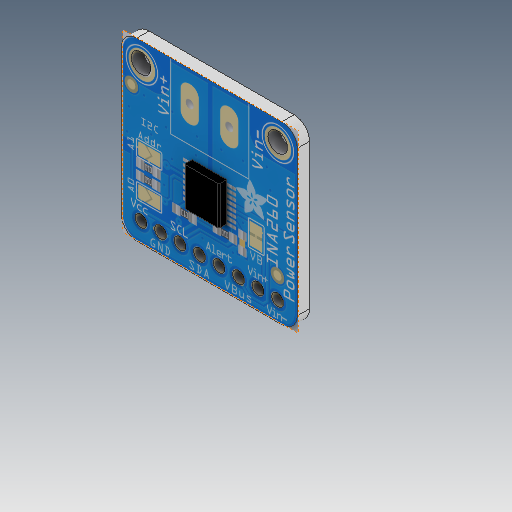
# Autodesk Inventor part: Adafruit_INA260
Saved by Autodesk Inventor 2020 (Build 240168000, 168)
## iProperties
Created: 2020-09-27
Part Number: Adafruit_INA260
Material: Generic
Document SubType Name: Modeling
Designer: DELL
Density: 1 g/cm^3
Appearance: Default
Author: DELL
Autodesk Inventor part; units mm, degrees
ref_plane "YZ Plane" through (0, 0, 0) normal (1, 0, 0) x (0, 1, 0)
ref_plane "XZ Plane" through (0, 0, 0) normal (0, 1, 0) x (-1, 0, 0)
ref_plane "XY Plane" through (0, 0, 0) normal (0, 0, 1) x (1, 0, 0)
sketch "Sketch1" plane through (0, 0, 0) normal (0, 0, 1) x (1, 0, 0)
  line L0 (11.43, -11.43) -> (-11.43, -11.43)
  line L1 (-11.43, -11.43) -> (-11.43, 11.43)
  line L2 (-11.43, 11.43) -> (11.43, 11.43)
  line L3 (11.43, 11.43) -> (11.43, -11.43)
  line L4 (11.43, -11.43) -> (-11.43, 11.43) construction
  line L5 (-11.43, -11.43) -> (11.43, 11.43) construction
  circle A0 centre (-8.89, 8.89) radius 1.27
  circle A1 centre (8.89, 8.89) radius 1.27
  line L6 (0, 11.43) -> (0, -11.43) construction
  circle A2 centre (-8.89, -8.89) radius 0.762
  circle A3 centre (-6.35, -8.89) radius 0.762
  circle A4 centre (-3.81, -8.89) radius 0.762
  circle A5 centre (-1.27, -8.89) radius 0.762
  circle A6 centre (1.27, -8.89) radius 0.762
  circle A7 centre (3.81, -8.89) radius 0.762
  circle A8 centre (6.35, -8.89) radius 0.762
  circle A9 centre (8.89, -8.89) radius 0.762
  point P0 (0, 0)
  dimension "d0" = 22.86
  dimension "d1" = 22.86
  dimension "d2" = 2.54
  dimension "d3" = 17.78
  dimension "d4" = 20.32
  dimension "d5" = 1.524
  dimension "d6" = 2.54
  dimension "d9" = 2.54
  constraints: 14 end point, 10 centre point, 4 midpoint, 2 horizontal, 2 parallel, 2 symmetric about line, 1 equal radius, 1 perpendicular, 14 other
  measures "d0" distance of L1.end L2.end
  measures "d1" distance of L0.end L1.end
  measures "d2" diameter of A0
  measures "d3" distance of A1.centre A0.centre
  measures "d4" distance from line of L0 A0.centre
  measures "d5" diameter of A2
  measures "d6" distance from line of L0 A2.centre
  measures "d9" distance of A2.centre A3.centre
extrude "Extrusion1" add sketch "Sketch1" along normal blind 1.6
fillet "Fillet1" radius 2 4 edges at (-11.43, 11.43, 0.8) (11.43, 11.43, 0.8) (11.43, -11.43, 0.8) (-11.43, -11.43, 0.8)
sketch "Sketch2" plane through (0, 0, 1.6) normal (0, 0, 1) x (1, 0, 0)
  line L0 (2.25, -3.68) -> (-2.25, -3.68)
  line L1 (-2.25, -3.68) -> (-2.25, 1.32)
  line L2 (-2.25, 1.32) -> (2.25, 1.32)
  line L3 (2.25, 1.32) -> (2.25, -3.68)
  line L4 (2.25, -3.68) -> (-2.25, 1.32) construction
  line L5 (-2.25, -3.68) -> (2.25, 1.32) construction
  line L6 (9.43, 11.43) -> (-9.43, 11.43) projected
  line L7 (-9.43, -11.43) -> (9.43, -11.43) projected
  point P0 (0, 0)
  point P1 (0, -1.18)
  point P2 (0, -1.18)
  dimension "d17" = 4.5
  dimension "d18" = 5
  dimension "d20" = 12.75
  constraints: 12 end point, 3 midpoint, 2 parallel, 1 horizontal, 1 perpendicular, 1 vertical alignment
  measures "d17" distance of L1.end L2.end
  measures "d18" distance of L2.end L0.start
  measures "d20" distance between parallel lines of L7 L2
extrude "Extrusion2" add sketch "Sketch2" along normal blind 1
chamfer "Chamfer1" distance 0.2 angle 45 2 edges at (-2.25, -1.18, 2.6) (2.25, -1.18, 2.6)
sketch "Sketch5" plane through (0, 0, 1.6) normal (0, 0, 1) x (1, 0, 0)
  line L0 (-11.3283, 11.4877) -> (11.6389, 11.4877) construction
  line L1 (11.6389, 11.4877) -> (11.6389, -11.3452) construction
  line L2 (11.6389, -11.3452) -> (-11.3283, -11.3452) construction
  line L3 (-11.3283, -11.3452) -> (-11.3283, 11.4877) construction
  point P0 (0, 0)
  constraints: 1 horizontal, 2 other
body "Solid1"
